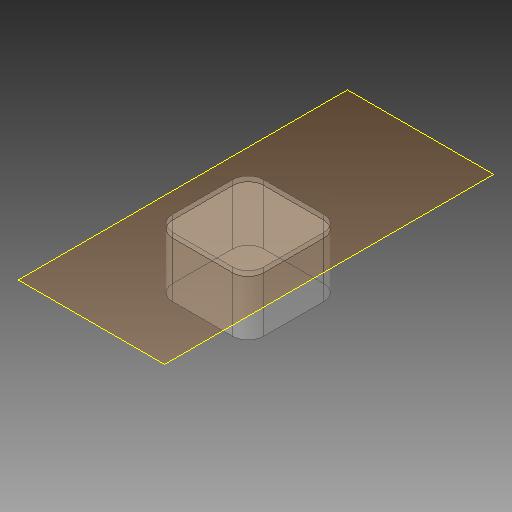
# Autodesk Inventor part: case
Saved by Autodesk Inventor 2019 (Build 230136000, 136)
## iProperties
Created: 2019-01-02
Part Number: case
Material: PET Plastic
Document SubType Name: Modeling
Designer: jmc
Density: 1.541 g/cm^3
Appearance: Polycarbonate - Clear
Author: jmc
Autodesk Inventor part; units mm, degrees
ref_plane "YZ Plane" through (0, 0, 0) normal (1, 0, 0) x (0, 1, 0)
ref_plane "XY Plane" through (0, 0, 0) normal (0, 0, 1) x (1, 0, 0)
sketch "Sketch1" plane through (0, 0, 0) normal (0, 1, 0) x (-1, 0, 0)
  line L0 (91.2118, 60) -> (91.2118, -60)
  arc A0 (60, -91.2118) -> (91.2118, -60) centre (60, -60) ccw
  arc A1 (-91.2118, -60) -> (-60, -91.2118) centre (-60, -60) ccw
  line L1 (-91.2118, -60) -> (-91.2118, 60)
  line L2 (-91.2118, 60) -> (-91.2118, 0)
  arc A2 (-60, 91.2118) -> (-91.2118, 60) centre (-60, 60) ccw
  line L3 (-60, 91.2118) -> (60, 91.2118)
  arc A3 (91.2118, 60) -> (60, 91.2118) centre (60, 60) ccw
  line L4 (60, -91.2118) -> (-60, -91.2118)
  line L5 (91.2118, 0) -> (-91.2118, 0) construction
  line L6 (0, -91.2118) -> (0, 91.2118) construction
  point P0 (0, 0)
  point P1 (0, 0)
  dimension "d15" = 120
  dimension "d17" = 120
  dimension "d18" = 120
  dimension "d19" = 120
  dimension "d20" = 31.2118
  constraints: 14 end point, 8 point on circle, 8 tangent, 5 midpoint, 4 centre point, 2 equal radius, 2 horizontal, 1 coincident, 1 parallel, 1 vertical
  measures "d15" distance of L0.start L0.end
  measures "d17" distance of L4.start L4.end
  measures "d18" distance of L1.start L1.end
  measures "d19" distance of L3.start L3.end
  measures "d20" radius of A0
ref_plane "Work Plane1" through (0, 110, 0) normal (0, 1, 0) x (-1, 0, 0)
extrude "Extrusion2" add sketch "Sketch1" along normal blind 120
split body "Split1" result two bodies by plane through (0, 110, 0) normal (0, 1, 0) first body at (-30.4039, 110.5, 0)
equation "\"d18\" = d17"
equation "\"d19\" = d18"
body "Solid3"
body "Solid4"
